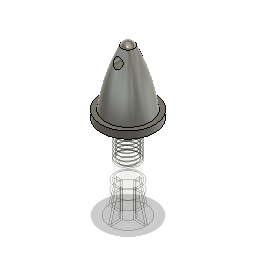
Minimal-Rotor-v24 (Autodesk Fusion 360 archive; units mm, degrees)
design "ROTOR SHAFT"
Autodesk Fusion 360 part; units mm, degrees
sketch "Sketch1" plane through (0, 0, 0) normal (0, 1, 0) x (1, 0, 0)
  circle A0 centre (0, 0) radius 2.5
  dimension "d1" = 5
  constraint coincident A0.centre origin
  measures "d1" diameter of A0
extrude "Extrude1" add sketch "Sketch1" along normal blind 14 makes body 1
thread "Thread1" "ISO Metric profile 5.0 M5x0.8 6g" major diameter 4.901 minor diameter 3.9895 pitch 0.8 angle 60 modelled right hand crest width 0.1157 on face at (2.4876, 9.3333, 0.2489) crest through (2.4505, -0.2, 0) on bodies 1
sketch "Sketch2" plane through (0, 0, 0) normal (0, -1, 0) x (1, 0, 0)
  spline S0 degree 3 poles (-1.1603, 1.6225) (-1.3903, 1.4937) (-1.5922, 1.3204) (-1.9269, 0.8987) (-2.0532, 0.6517) (-2.209, 0.1131) (-2.233, -0.1744) (-2.1704, -0.754) (-2.0801, -1.0399) (-1.8392, -1.4841) (-1.7158, -1.6529) (-1.4249, -1.9579) (-1.2576, -2.0917) (-1.0751, -2.2021) knots 0 0 0 0 0.079059 0.079059 0.16138 0.16138 0.246963 0.246963 0.335805 0.335805 0.398048 0.398048 0.461789 0.461789 0.461789 0.461789
  arc A0 (-1.0751, -2.2021) -> (1.0751, -2.2021) centre (0, 0) ccw
  spline S1 degree 3 poles (1.0751, -2.2021) (1.3425, -2.0404) (1.5763, -1.8288) (1.9414, -1.3357) (2.0726, -1.0614) (2.2176, -0.4881) (2.2341, -0.1957) (2.1537, 0.3677) (2.0617, 0.6338) (1.8279, 1.0317) (1.7152, 1.1764) (1.4579, 1.4285) (1.3153, 1.5357) (1.1603, 1.6225) knots 0 0 0 0 0.093745 0.093745 0.184219 0.184219 0.271423 0.271423 0.355353 0.355353 0.410323 0.410323 0.463803 0.463803 0.463803 0.463803
  arc A1 (1.1603, 1.6225) -> (-1.1603, 1.6225) centre (0, 0) ccw
  circle A2 centre (0, 0) radius 2.5
  dimension "d4" = 5
  constraint concentric A0 A2
  measures "d4" diameter of A2
extrude "Extrude2" add sketch "Sketch2" along normal blind 4 contours S0 A0 S1 A1 | A2 bodies 1
sketch "Sketch4" plane through (0, 0, 0) normal (1, 0, 0) x (0, 0, -1)
  line L0 (0, -4) -> (2.885, -4)
  line L1 (2.885, -4) -> (2.885, -6)
  line L2 (2.885, -6) -> (4.15, -11)
  line L3 (4.15, -11) -> (0, -11)
  line L4 (0, -11) -> (0, -4)
  dimension "d7" = 2
  dimension "d8" = 5
  dimension "d9" = 4.15
  dimension "d10" = 4
  dimension "d11" = 2.885
  constraint horizontal L0
  constraint perpendicular L0 L1
  constraint perpendicular L1 L3
  constraint vertical origin L0.start
  constraint vertical L4
  measures "d7" distance of L0.end L1.end
  measures "d8" vertical distance of L1.end L2.end
  measures "d9" distance of L2.end L3.end
  measures "d10" vertical distance of origin L0.start
  measures "d11" distance of L0.start L1
revolve "Revolve1" add sketch "Sketch4" angle 360 about axis through (0, 1.75, 0) along (0, 1, 0) bodies 1
copy_body "Body->Comp1" bodies 1 removing the originals makes body 2 in component "SHAFT"
sketch "Sketch5" plane through (0, -11, 0) normal (0, -1, 0) x (1, 0, 0)
  circle A0 centre (0, 0) radius 4.15
  circle A1 centre (0, 0) radius 1.45
  dimension "d13" = 2.9
  constraint concentric A0 A1
  measures "d13" diameter of A1
extrude "Extrude1'" cut sketch "Sketch5" against normal blind 10.5 contours A1 bodies 2 in component "SHAFT"
sketch "Sketch6" plane through (0, -11, 0) normal (0, -1, 0) x (1, 0, 0)
  circle A0 centre (0, 0) radius 1.45
  circle A1 centre (0, 0) radius 4.15
  line L0 (-0.25, 1.4283) -> (0.25, 1.4283)
  line L1 (0.25, 1.4283) -> (0.25, 5.1127)
  line L2 (0.25, 5.1127) -> (-0.25, 5.1127)
  line L3 (-0.25, 5.1127) -> (-0.25, 1.4283)
  line L4 (0.25, -1.4283) -> (-0.25, -1.4283)
  line L5 (-0.25, -1.4283) -> (-0.25, -5.616)
  line L6 (-0.25, -5.616) -> (0.25, -5.616)
  line L7 (0.25, -5.616) -> (0.25, -1.4283)
  line L8 (5.163, 0.25) -> (1.4283, 0.25)
  line L9 (1.4283, 0.25) -> (1.4283, -0.25)
  line L10 (1.4283, -0.25) -> (5.163, -0.25)
  line L11 (5.163, -0.25) -> (5.163, 0.25)
  line L12 (-1.4283, 0.25) -> (-6.3952, 0.25)
  line L13 (-6.3952, 0.25) -> (-6.3952, -0.25)
  line L14 (-6.3952, -0.25) -> (-1.4283, -0.25)
  line L15 (-1.4283, -0.25) -> (-1.4283, 0.25)
  dimension "d16" = 0.25
  dimension "d17" = 0.5
  dimension "d18" = 0.25
  dimension "d19" = 0.5
  constraint horizontal L0
  constraint vertical L1
  constraint horizontal L2
  constraint vertical L3
  constraint coincident A0 L0.start
  constraint horizontal L4
  constraint vertical L5
  constraint horizontal L6
  constraint vertical L7
  constraint coincident A0 L4.start
  constraint collinear L1 L7
  constraint collinear L3 L5
  constraint horizontal L8
  constraint vertical L9
  constraint horizontal L10
  constraint vertical L11
  constraint coincident A0 L9.end
  constraint horizontal L12
  constraint vertical L13
  constraint horizontal L14
  constraint vertical L15
  constraint coincident A0 L12.start
  constraint collinear L8 L12
  constraint collinear L10 L14
  measures "d16" horizontal distance of A0.centre L0.start
  measures "d17" distance of L1.end L2.end
  measures "d18" vertical distance of A0.centre L8.end
  measures "d19" distance of L8.start L10.end
extrude "Extrude2'" cut sketch "Sketch6" against normal blind 6 contours A0 A1 L8 L10 | A0 A1 L1 L3 | A0 A1 L5 L7 | A0 A1 L12 L14 bodies 2 in component "SHAFT"
sketch "Sketch1 (2)" plane through (0, 0, 0) normal (0, 0, 1) x (1, 0, 0) in component "ROTOR TOP"
  line L0 (0, 8.1239) -> (-6, 8.1239)
  line L1 (-6, 8.1239) -> (-6, 9.7239)
  line L2 (-6, 9.7239) -> (-5, 9.7239)
  circle A0 through (0, 24.6239, 0) (0, 20.1239, 2.5981) (0, 20.1239, -2.5981)
  circle A1 centre (0, 21.6239) radius 1.5
  arc A2 (-1.3649, 22.2459) -> (-5, 9.7239) centre (39.6733, 3.5442) ccw
  line L3 (0, 23.1239) -> (0, 8.1239)
  line L4 (0, 13.9817) -> (-2.5479, 13.9817)
  line L5 (-2.5479, 13.9817) -> (-2.5479, 8.1239)
  point P0 (0, 23.1239)
  dimension "d22" = 6
  dimension "d23" = 1.6
  dimension "d24" = 5
  dimension "d25" = 15
  dimension "d26" = 3
  dimension "d27" = 13.5
  dimension "d29" = 45.0987
  constraint horizontal L0
  constraint perpendicular L0 L1
  constraint vertical origin L0.start
  constraint perpendicular L1 L2
  constraint tangent A1 A2
  constraint coincident A1 A2.start
  constraint coincident P0 L3.start
  constraint perpendicular L0 L3
  constraint coincident L3 L4.start
  constraint perpendicular L3 L4
  constraint coincident L0 L5.end
  constraint perpendicular L0 L5
  measures "d22" distance of L0.start L0.end
  measures "d23" distance of L0.end L1.end
  measures "d24" horizontal distance of origin L2.end
  measures "d25" distance of L0.start P0
  measures "d26" diameter of A1
  measures "d27" distance of L0.start A1.centre
  measures "d29" radius of A2
revolve "Revolve1'" add sketch "Sketch1 (2)" angle 360 about axis through (0, 1.75, 0) along (0, 1, 0) separate body contours L0 L1 L2 A1 A2 L3 L4 L5 | A1 L3 picked at (-0.4823, 21.188) makes body 3 in component "ROTOR TOP"
sketch "Sketch2 (2)" plane through (0, 0, 0) normal (0, 0, 1) x (1, 0, 0) in component "ROTOR TOP"
  circle A0 centre (0, 19.8739) radius 1
  line L0 (6, 8.1239) -> (-6, 8.1239)
  dimension "d30" = 2
  dimension "d31" = 11.75
  measures "d30" diameter of A0
  measures "d31" distance of A0.centre L0
extrude "Extrude1''" cut sketch "Sketch2 (2)" along normal blind 12 and the other way blind 10 bodies 3 in component "ROTOR TOP"
component "SHAFT" placed x (1, 0, 0) y (0, 1, 0) z (0, 0, 1) at (0, 0, 0)
component "ROTOR TOP" placed x (1, 0, 0) y (0, 1, 0) z (0, 0, 1) at (0, 0, 0)
equation "d11 = ( 5.77 / 2 ) * 1 mm"
equation "d27 = 15 mm - 1.5 mm"
